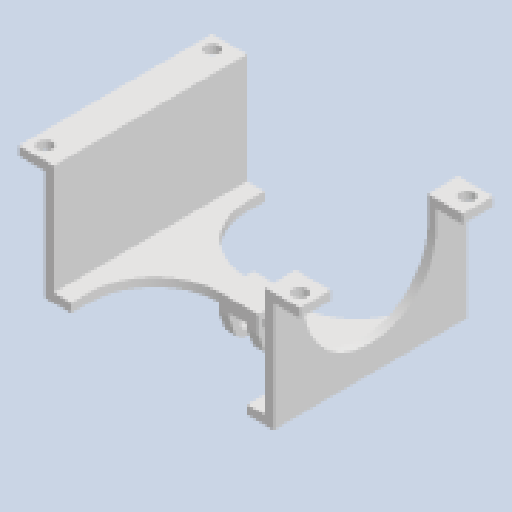
# Autodesk Inventor part: carlig
Saved by Autodesk Inventor 2025.2 (Build 292293000, 293)
## iProperties
Created: 2025-04-05
Part Number: carlig
Material: Generic
Document SubType Name: Modeling
Designer: mirewn
Density: 1 g/cm^3
Appearance: Default
Author: mirewn
Autodesk Inventor part; units mm, degrees
ref_plane "YZ Plane" through (0, 0, 0) normal (1, 0, 0) x (0, 1, 0)
ref_plane "XZ Plane" through (0, 0, 0) normal (0, 1, 0) x (-1, 0, 0)
ref_plane "XY Plane" through (0, 0, 0) normal (0, 0, 1) x (1, 0, 0)
sketch "Sketch1" plane through (0, 0, 0) normal (0, 0, 1) x (1, 0, 0)
  line L0 (0, 0) -> (-26, 0)
  line L1 (-26, 0) -> (-26, 25)
  line L2 (-26, 25) -> (-32, 25)
  line L3 (-32, 25) -> (-32, 27)
  line L4 (-32, 27) -> (-24, 27)
  line L5 (-24, 27) -> (-24, 2)
  line L6 (-24, 2) -> (0, 2)
  line L7 (0, 0) -> (0, 2) construction
  line L8 (0, 0) -> (26, 0)
  line L9 (26, 0) -> (26, 25)
  line L10 (26, 25) -> (32, 25)
  line L11 (32, 25) -> (32, 27)
  line L12 (32, 27) -> (24, 27)
  line L13 (24, 27) -> (24, 2)
  line L14 (24, 2) -> (0, 2)
  point P0 (29, 25)
  point P1 (-28, 27)
  point P2 (-29, 25)
  dimension "d0" = 25
  dimension "d1" = 6
  dimension "d4" = 2
  dimension "d5" = 2
  dimension "d18" = 2
  dimension "d19" = 29
  constraints: 30 end point, 6 symmetric about line, 3 vertical, 2 horizontal, 2 midpoint, 2 perpendicular, 1 parallel
  measures "d0" distance of L0.end L1.end
  measures "d1" distance of L1.end L2.end
  measures "d4" distance between parallel lines of L2 L4
  measures "d5" distance between parallel lines of L0 L6
  measures "d18" distance between parallel lines of L1 L5
  measures "d19" horizontal distance of L0.start point (-29, 25)
extrude "Extrusion1" add sketch "Sketch1" along normal blind 44
sketch "Sketch2" plane through (-32, 27, 0) normal (0, 1, 0) x (1, 0, 0)
  line L0 (32, 0) -> (32, -44) construction
  line L1 (61, -41) -> (3, -41) construction
  line L2 (3, -41) -> (3, -3) construction
  line L3 (3, -3) -> (61, -3) construction
  line L4 (61, -3) -> (61, -41) construction
  line L5 (61, -41) -> (3, -3) construction
  line L6 (3, -41) -> (61, -3) construction
  point P0 (32, -22)
  point P1 (64, -44)
  dimension "d8" = 38
  dimension "d9" = 58
  constraints: 14 end point, 4 coincident, 3 midpoint, 2 parallel, 1 horizontal, 1 horizontal alignment, 1 perpendicular, 1 vertical
  measures "d8" distance of L1.end L2.end
  measures "d9" distance of L2.end L3.end
hole "Hole1" at (-29, 27, 41) at (-29, 27, 3) at (29, 27, 41) at (29, 27, 3) direction (0, -1, 0) diameter 3.2 end through all
sketch "Sketch3" plane through (32, 25, 0) normal (1, 0, 0) x (0, 0, -1)
  line L0 (0, 2) -> (-44, 2) construction
  line L1 (-22, 2) -> (-22, -19) construction
  line L2 (0, -23) -> (-44, -23) construction
  line L3 (-7, 2) -> (-7, -19)
  line L4 (-7, -19) -> (-22, -19)
  line L5 (-7, 2) -> (-37, 2)
  line L6 (-37, 2) -> (-37, -19)
  line L7 (-37, -19) -> (-22, -19)
  point P0 (0, -25)
  dimension "d20" = 21
  dimension "d21" = 15
  dimension "d22" = 15
  constraints: 12 end point, 3 perpendicular, 2 point on line, 2 vertical, 1 midpoint
  measures "d20" distance of L1.start L1.end
  measures "d21" distance between parallel lines of L1 L3
  measures "d22" distance of L6.end L1.end
extrude "Extrusion2" cut sketch "Sketch3" against normal up to surface (56 mm away)
sketch "Sketch4" plane through (-26, 0, 0) normal (0, -1, 0) x (1, 0, 0)
  line L0 (0, 0) -> (52, 0) projected
  line L1 (52, 0) -> (46, 0)
  line L2 (46, 0) -> (46, 19)
  line L3 (50, 44) -> (2, 44) projected
  line L4 (46, 19) -> (6, 19)
  line L5 (6, 19) -> (6, 0)
  line L6 (52, 0) -> (52, 44) construction
  line L7 (52, 22) -> (0, 22) construction
  line L8 (0, 0) -> (0, 44) construction
  line L9 (46, 0) -> (6, 0) construction
  line L10 (46, 44) -> (46, 25)
  line L11 (46, 25) -> (6, 25)
  line L12 (6, 25) -> (6, 44)
  line L13 (46, 44) -> (6, 44) construction
  point P0 (26, 0)
  point P1 (26, 44)
  point P2 (6, 0)
  dimension "d25" = 6
  dimension "d26" = 19
  dimension "d27" = 40
  constraints: 20 end point, 5 symmetric about line, 2 midpoint, 2 perpendicular, 2 point on line, 1 collinear, 1 parallel
  measures "d25" distance of L0.end L1.end
  measures "d26" distance of L1.end L2.end
  measures "d27" distance of L2.end L4.end
extrude "Extrusion3" cut sketch "Sketch4" against normal blind 10
sketch "Sketch5" plane through (0, 0, 0) normal (1, 0, 0) x (0, 1, 0)
  line L0 (0, 0) -> (0, 44) construction
  line L1 (0, 22) -> (-30, 22) construction
  line L2 (3, 18) -> (-1, 18)
  line L3 (-1, 22) -> (-1, 26)
  line L4 (-1, 26) -> (3, 26)
  line L5 (3, 26) -> (3, 18)
  line L6 (3, 18) -> (-1, 26) construction
  line L7 (-1, 18) -> (3, 26) construction
  circle A0 centre (-3.5, 22) radius 1.6
  arc A1 (-4.4519, 24.845) -> (-4.4519, 19.155) centre (-3.5, 22) ccw
  line L8 (-1, 18) -> (-4.4519, 19.155)
  line L9 (-1, 26) -> (-4.4519, 24.845)
  circle A2 centre (-3.5, 22) radius 3
  line L10 (0, 0) -> (0, 44) projected
  line L11 (0, 26) -> (0, 18)
  point P0 (1, 22)
  dimension "d30" = 3.2
  dimension "d31" = 6
  dimension "d32" = 4.5
  constraints: 20 end point, 6 point on line, 3 centre point, 3 midpoint, 3 tangent, 2 coincident, 2 horizontal, 2 parallel, 2 point on circle, 1 perpendicular
  measures "d30" diameter of A0
  measures "d31" diameter of A1
  measures "d32" distance of A0.centre point (1, 22)
extrude "Extrusion4" add sketch "Sketch5" along normal mid plane 9
extrude "Extrusion5" cut sketch "Sketch5" along normal mid plane 4 contours L2 L8 A2 L3 L4 L10 | A1 A2 | L3 A2 L9
fillet "Fillet1" radius 15 6 edges at (20, 1, 25) (20, 1, 19) (-20, 1, 25) (-20, 1, 19) (25, 6, 37) (25, 6, 7)
body "Solid1"
